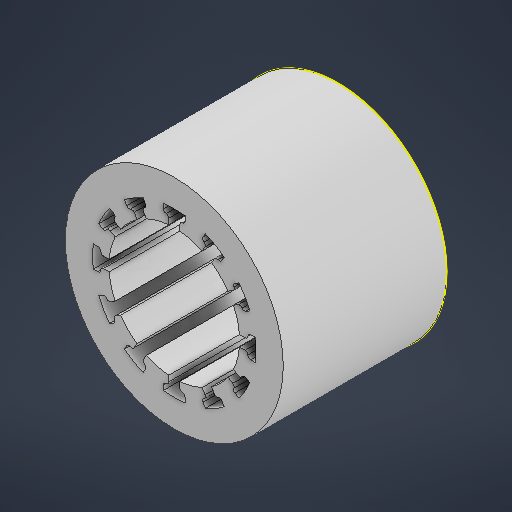
# Autodesk Inventor part: СИСЬКА
Saved by Autodesk Inventor 2025 (Build 290162000, 162)
## iProperties
Created: 2025-10-03
Part Number: СИСЬКА
Material: Типовые
Document SubType Name: Modeling
Designer: Phantom
Density: 1 g/cm^3
Appearance: По умолчанию
Author: Phantom
Autodesk Inventor part; units mm, degrees
ref_plane "YZ Plane" through (0, 0, 0) normal (1, 0, 0) x (0, 1, 0)
ref_plane "XZ Plane" through (0, 0, 0) normal (0, 1, 0) x (-1, 0, 0)
ref_plane "XY Plane" through (0, 0, 0) normal (0, 0, 1) x (1, 0, 0)
sketch "Эскиз1" plane through (0, 0, 0) normal (0, 0, 1) x (1, 0, 0)
  line L0 (-10.0069, -9.9098) -> (-10.0069, 10.0902)
  line L1 (-10.0069, 10.0902) -> (9.9931, 10.0902)
  line L2 (9.9931, 10.0902) -> (9.9931, -9.9098)
  line L3 (9.9931, -9.9098) -> (-10.0069, -9.9098)
  arc A0 (15.9207, 25.1962) -> (15.3056, 28.1887) centre (14.3486, 26.4325) ccw
  line L4 (10.8274, 18.7196) -> (15.9207, 25.1962)
  arc A1 (8.4102, 18.1432) -> (10.8274, 18.7196) centre (9.2553, 19.9559) ccw
  arc A2 (8.4102, 18.1432) -> (6.3595, 18.9642) centre (-0.0069, 0.0902) ccw
  arc A3 (5.0078, 21.0494) -> (6.3595, 18.9642) centre (6.9987, 20.8593) ccw
  line L5 (5.791, 29.2515) -> (5.0078, 21.0494)
  arc A4 (8.3012, 30.9928) -> (5.791, 29.2515) centre (7.7819, 29.0614) ccw
  arc A5 (8.3012, 30.9928) -> (-2.3164, 32.0067) centre (-0.0069, 0.0902) ccw
  arc A6 (-0.1811, 29.8218) -> (-2.3164, 32.0067) centre (-2.1721, 30.0119) ccw
  line L6 (-0.9643, 21.6197) -> (-0.1811, 29.8218)
  arc A7 (-2.6862, 19.828) -> (-0.9643, 21.6197) centre (-2.9553, 21.8098) ccw
  arc A8 (-2.6862, 19.828) -> (-4.8552, 19.4099) centre (-0.0069, 0.0902) ccw
  arc A9 (-7.1197, 20.4333) -> (-4.8552, 19.4099) centre (-5.342, 21.3498) ccw
  line L7 (-10.8952, 27.7568) -> (-7.1197, 20.4333)
  arc A10 (-9.7249, 30.5788) -> (-10.8952, 27.7568) centre (-9.1176, 28.6733) ccw
  arc A11 (-9.7249, 30.5788) -> (-19.2052, 25.6914) centre (-0.0069, 0.0902) ccw
  arc A12 (-16.2276, 25.0078) -> (-19.2052, 25.6914) centre (-18.0053, 24.0914) ccw
  line L8 (-12.4521, 17.6843) -> (-16.2276, 25.0078)
  arc A13 (-12.932, 15.2461) -> (-12.4521, 17.6843) centre (-14.2297, 16.7678) ccw
  arc A14 (-12.932, 15.2461) -> (-14.5306, 13.7218) centre (-0.0069, 0.0902) ccw
  arc A15 (-16.9889, 13.3584) -> (-14.5306, 13.7218) centre (-15.9889, 15.0905) ccw
  line L9 (-24.1245, 17.4781) -> (-16.9889, 13.3584)
  arc A16 (-24.6657, 20.4849) -> (-24.1245, 17.4781) centre (-23.1245, 19.2102) ccw
  arc A17 (-24.6657, 20.4849) -> (-29.9986, 11.2479) centre (-0.0069, 0.0902) ccw
  arc A18 (-27.1241, 12.2826) -> (-29.9986, 11.2479) centre (-28.1241, 10.5506) ccw
  line L10 (-19.9885, 8.1629) -> (-27.1241, 12.2826)
  arc A19 (-19.0741, 5.8523) -> (-19.9885, 8.1629) centre (-20.9885, 6.4309) ccw
  arc A20 (-19.0741, 5.8523) -> (-19.5948, 3.7057) centre (-0.0069, 0.0902) ccw
  arc A21 (-21.4664, 2.0709) -> (-19.5948, 3.7057) centre (-21.5616, 4.0687) ccw
  line L11 (-29.6965, 1.6789) -> (-21.4664, 2.0709)
  arc A22 (-31.7774, 3.9157) -> (-29.6965, 1.6789) centre (-29.7917, 3.6766) ccw
  arc A23 (-31.7774, 3.9157) -> (-31.2699, -6.7381) centre (-0.0069, 0.0902) ccw
  arc A24 (-29.4111, -4.3136) -> (-31.2699, -6.7381) centre (-29.3159, -6.3113) ccw
  line L12 (-21.181, -3.9215) -> (-29.4111, -4.3136)
  arc A25 (-19.1625, -5.3709) -> (-21.181, -3.9215) centre (-21.0858, -5.9193) ccw
  arc A26 (-19.1625, -5.3709) -> (-18.44, -7.4583) centre (-0.0069, 0.0902) ccw
  arc A27 (-19.1307, -9.8454) -> (-18.44, -7.4583) centre (-20.2908, -8.2163) ccw
  line L13 (-25.8424, -14.6248) -> (-19.1307, -9.8454)
  arc A28 (-28.8022, -13.868) -> (-25.8424, -14.6248) centre (-27.0025, -12.9956) ccw
  arc A29 (-28.8022, -13.868) -> (-22.6154, -22.5562) centre (-0.0069, 0.0902) ccw
  arc A30 (-22.3624, -19.5116) -> (-22.6154, -22.5562) centre (-21.2023, -21.1408) ccw
  line L14 (-15.6508, -14.7323) -> (-22.3624, -19.5116)
  arc A31 (-13.1691, -14.8603) -> (-15.6508, -14.7323) centre (-14.4907, -16.3614) ccw
  arc A32 (-13.1691, -14.8603) -> (-11.4328, -16.2257) centre (-0.0069, 0.0902) ccw
  arc A33 (-10.7233, -18.6073) -> (-11.4328, -16.2257) centre (-12.58, -17.864) ccw
  line L15 (-13.7856, -26.2565) -> (-10.7233, -18.6073)
  arc A34 (-16.6847, -27.2201) -> (-13.7856, -26.2565) centre (-15.6423, -25.5132) ccw
  arc A35 (-16.6847, -27.2201) -> (-6.7828, -31.1842) centre (-0.0069, 0.0902) ccw
  arc A36 (-8.2161, -28.4862) -> (-6.7828, -31.1842) centre (-6.3593, -29.2296) ccw
  line L16 (-5.1538, -20.837) -> (-8.2161, -28.4862)
  arc A37 (-2.9968, -19.603) -> (-5.1538, -20.837) centre (-3.297, -21.5803) ccw
  arc A38 (-2.9968, -19.603) -> (-0.7979, -19.813) centre (-0.0069, 0.0902) ccw
  arc A39 (1.0865, -21.4329) -> (-0.7979, -19.813) centre (-0.8773, -21.8114) ccw
  line L17 (2.6459, -29.5234) -> (1.0865, -21.4329)
  arc A40 (0.7279, -31.9014) -> (2.6459, -29.5234) centre (0.682, -29.9019) ccw
  arc A41 (0.7279, -31.9014) -> (11.201, -29.8829) centre (-0.0069, 0.0902) ccw
  arc A42 (8.5367, -28.3881) -> (11.201, -29.8829) centre (10.5006, -28.0096) ccw
  line L18 (6.9789, -20.3054) -> (8.5367, -28.3881)
  arc A43 (8.1187, -18.1045) -> (6.9789, -20.3054) centre (8.9427, -19.9268) ccw
  arc A44 (8.1187, -18.1045) -> (10.086, -17.0832) centre (-0.3176, 0.5517) ccw
  arc A45 (12.5497, -17.4256) -> (10.086, -17.0832) centre (11.1023, -18.8058) ccw
  line L19 (18.2351, -23.3882) -> (12.5497, -17.4256)
  arc A46 (17.9072, -26.4256) -> (18.2351, -23.3882) centre (16.7876, -24.7684) ccw
  arc A47 (17.9072, -26.4256) -> (25.6265, -19.0653) centre (-0.0069, 0.0902) ccw
  arc A48 (22.5769, -19.2482) -> (25.6265, -19.0653) centre (24.0244, -17.8681) ccw
  line L20 (16.8911, -13.2851) -> (22.5769, -19.2482)
  arc A49 (16.6646, -10.8104) -> (16.8911, -13.2851) centre (18.3385, -11.9049) ccw
  arc A50 (16.6646, -10.8104) -> (17.769, -8.8975) centre (-0.0069, 0.0902) ccw
  arc A51 (20.0254, -7.8563) -> (17.769, -8.8975) centre (19.5539, -9.7999) ccw
  line L21 (28.0326, -9.7988) -> (20.0254, -7.8563)
  arc A52 (29.3989, -12.5312) -> (28.0326, -9.7988) centre (27.5611, -11.7424) ccw
  arc A53 (29.3989, -12.5312) -> (31.9135, -2.166) centre (-0.0069, 0.0902) ccw
  arc A54 (29.447, -3.9686) -> (31.9135, -2.166) centre (29.9185, -2.025) ccw
  line L22 (21.4398, -2.0261) -> (29.447, -3.9686)
  arc A55 (19.9114, -0.0667) -> (21.4398, -2.0261) centre (21.9113, -0.0825) ccw
  arc A56 (19.9114, -0.0667) -> (19.8062, 2.1397) centre (-0.0069, 0.0902) ccw
  arc A57 (21.1415, 4.2355) -> (19.8062, 2.1397) centre (21.7956, 2.3455) ccw
  line L23 (28.9278, 6.9303) -> (21.1415, 4.2355)
  arc A58 (31.5545, 5.3703) -> (28.9278, 6.9303) centre (29.5819, 5.0403) ccw
  arc A59 (31.5545, 5.3703) -> (23.2125, 22.1098) centre (-0.0069, 0.0902) ccw
  arc A60 (26.9459, 12.7815) -> (28.2217, 15.1615) centre (26.2834, 14.6686) ccw
  line L24 (19.1717, 10.0522) -> (26.9459, 12.7815)
  arc A61 (16.8229, 10.8638) -> (19.1717, 10.0522) centre (18.5092, 11.9393) ccw
  arc A62 (16.8229, 10.8638) -> (15.5337, 12.6575) centre (0.0291, 0.1528) ccw
  arc A63 (15.5129, 15.1424) -> (15.5337, 12.6575) centre (17.0905, 13.913) ccw
  line L25 (20.5775, 21.6415) -> (15.5129, 15.1424)
  arc A64 (23.2125, 22.1098) -> (20.5775, 21.6415) centre (22.155, 20.4122) ccw
  arc A65 (23.2125, 22.1098) -> (15.3056, 28.1887) centre (-0.0069, 0.0902) ccw
  arc A66 (8.4102, 18.1432) -> (6.3595, 18.9642) centre (-0.0069, 0.0902) ccw
  arc A67 (8.4102, 18.1432) -> (10.8274, 18.7196) centre (9.2553, 19.9559) ccw
  line L26 (10.8274, 18.7196) -> (15.9207, 25.1962)
  arc A68 (15.9207, 25.1962) -> (15.3056, 28.1887) centre (14.3486, 26.4325) ccw
  arc A69 (15.3056, 28.1887) -> (8.3012, 30.9928) centre (-0.0069, 0.0902) ccw
  arc A70 (8.3012, 30.9928) -> (5.791, 29.2515) centre (7.7819, 29.0614) ccw
  line L27 (5.791, 29.2515) -> (5.0078, 21.0494)
  arc A71 (5.0078, 21.0494) -> (6.3595, 18.9642) centre (6.9987, 20.8593) ccw
  line L28 (-0.9643, 21.6197) -> (-0.1811, 29.8218)
  arc A72 (-0.1811, 29.8218) -> (-2.3164, 32.0067) centre (-2.1721, 30.0119) ccw
  arc A73 (-2.3164, 32.0067) -> (-9.7249, 30.5788) centre (-0.0069, 0.0902) ccw
  arc A74 (-9.7249, 30.5788) -> (-10.8952, 27.7568) centre (-9.1176, 28.6733) ccw
  line L29 (-10.8952, 27.7568) -> (-7.1197, 20.4333)
  arc A75 (-7.1197, 20.4333) -> (-4.8552, 19.4099) centre (-5.342, 21.3498) ccw
  arc A76 (-2.6862, 19.828) -> (-4.8552, 19.4099) centre (-0.0069, 0.0902) ccw
  arc A77 (-2.6862, 19.828) -> (-0.9643, 21.6197) centre (-2.9553, 21.8098) ccw
  arc A78 (-12.932, 15.2461) -> (-14.5306, 13.7218) centre (-0.0069, 0.0902) ccw
  arc A79 (-12.932, 15.2461) -> (-12.4521, 17.6843) centre (-14.2297, 16.7678) ccw
  line L30 (-12.4521, 17.6843) -> (-16.2276, 25.0078)
  arc A80 (-16.2276, 25.0078) -> (-19.2052, 25.6914) centre (-18.0053, 24.0914) ccw
  arc A81 (-19.2052, 25.6914) -> (-24.6657, 20.4849) centre (-0.0069, 0.0902) ccw
  arc A82 (-24.6657, 20.4849) -> (-24.1245, 17.4781) centre (-23.1245, 19.2102) ccw
  line L31 (-24.1245, 17.4781) -> (-16.9889, 13.3584)
  arc A83 (-16.9889, 13.3584) -> (-14.5306, 13.7218) centre (-15.9889, 15.0905) ccw
  arc A84 (-29.9986, 11.2479) -> (-31.7774, 3.9157) centre (-0.0069, 0.0902) ccw
  arc A85 (-31.7774, 3.9157) -> (-29.6965, 1.6789) centre (-29.7917, 3.6766) ccw
  line L32 (-29.6965, 1.6789) -> (-21.4664, 2.0709)
  arc A86 (-21.4664, 2.0709) -> (-19.5948, 3.7057) centre (-21.5616, 4.0687) ccw
  arc A87 (-19.0741, 5.8523) -> (-19.5948, 3.7057) centre (-0.0069, 0.0902) ccw
  arc A88 (-19.0741, 5.8523) -> (-19.9885, 8.1629) centre (-20.9885, 6.4309) ccw
  line L33 (-19.9885, 8.1629) -> (-27.1241, 12.2826)
  arc A89 (-27.1241, 12.2826) -> (-29.9986, 11.2479) centre (-28.1241, 10.5506) ccw
  arc A90 (-31.2699, -6.7381) -> (-28.8022, -13.868) centre (-0.0069, 0.0902) ccw
  arc A91 (-28.8022, -13.868) -> (-25.8424, -14.6248) centre (-27.0025, -12.9956) ccw
  line L34 (-25.8424, -14.6248) -> (-19.1307, -9.8454)
  arc A92 (-19.1307, -9.8454) -> (-18.44, -7.4583) centre (-20.2908, -8.2163) ccw
  arc A93 (-19.1625, -5.3709) -> (-18.44, -7.4583) centre (-0.0069, 0.0902) ccw
  arc A94 (-19.1625, -5.3709) -> (-21.181, -3.9215) centre (-21.0858, -5.9193) ccw
  line L35 (-21.181, -3.9215) -> (-29.4111, -4.3136)
  arc A95 (-29.4111, -4.3136) -> (-31.2699, -6.7381) centre (-29.3159, -6.3113) ccw
  arc A96 (-6.7828, -31.1842) -> (0.7279, -31.9014) centre (-0.0069, 0.0902) ccw
  arc A97 (0.7279, -31.9014) -> (2.6459, -29.5234) centre (0.682, -29.9019) ccw
  line L36 (2.6459, -29.5234) -> (1.0865, -21.4329)
  arc A98 (1.0865, -21.4329) -> (-0.7979, -19.813) centre (-0.8773, -21.8114) ccw
  arc A99 (-2.9968, -19.603) -> (-0.7979, -19.813) centre (-0.0069, 0.0902) ccw
  arc A100 (-2.9968, -19.603) -> (-5.1538, -20.837) centre (-3.297, -21.5803) ccw
  line L37 (-5.1538, -20.837) -> (-8.2161, -28.4862)
  arc A101 (-8.2161, -28.4862) -> (-6.7828, -31.1842) centre (-6.3593, -29.2296) ccw
  arc A102 (11.201, -29.8829) -> (17.9072, -26.4256) centre (-0.0069, 0.0902) ccw
  arc A103 (17.9072, -26.4256) -> (18.2351, -23.3882) centre (16.7876, -24.7684) ccw
  line L38 (18.2351, -23.3882) -> (12.5497, -17.4256)
  arc A104 (12.5497, -17.4256) -> (10.086, -17.0832) centre (11.1023, -18.8058) ccw
  arc A105 (8.1187, -18.1045) -> (10.086, -17.0832) centre (-0.3176, 0.5517) ccw
  arc A106 (8.1187, -18.1045) -> (6.9789, -20.3054) centre (8.9427, -19.9268) ccw
  line L39 (6.9789, -20.3054) -> (8.5367, -28.3881)
  arc A107 (8.5367, -28.3881) -> (11.201, -29.8829) centre (10.5006, -28.0096) ccw
  arc A108 (-22.6154, -22.5562) -> (-16.6847, -27.2201) centre (-0.0069, 0.0902) ccw
  arc A109 (-16.6847, -27.2201) -> (-13.7856, -26.2565) centre (-15.6423, -25.5132) ccw
  line L40 (-13.7856, -26.2565) -> (-10.7233, -18.6073)
  arc A110 (-10.7233, -18.6073) -> (-11.4328, -16.2257) centre (-12.58, -17.864) ccw
  arc A111 (-13.1691, -14.8603) -> (-11.4328, -16.2257) centre (-0.0069, 0.0902) ccw
  arc A112 (-13.1691, -14.8603) -> (-15.6508, -14.7323) centre (-14.4907, -16.3614) ccw
  line L41 (-15.6508, -14.7323) -> (-22.3624, -19.5116)
  arc A113 (-22.3624, -19.5116) -> (-22.6154, -22.5562) centre (-21.2023, -21.1408) ccw
  arc A114 (16.6646, -10.8104) -> (17.769, -8.8975) centre (-0.0069, 0.0902) ccw
  arc A115 (16.6646, -10.8104) -> (16.8911, -13.2851) centre (18.3385, -11.9049) ccw
  line L42 (16.8911, -13.2851) -> (22.5769, -19.2482)
  arc A116 (22.5769, -19.2482) -> (25.6265, -19.0653) centre (24.0244, -17.8681) ccw
  arc A117 (25.6265, -19.0653) -> (29.3989, -12.5312) centre (-0.0069, 0.0902) ccw
  arc A118 (29.3989, -12.5312) -> (28.0326, -9.7988) centre (27.5611, -11.7424) ccw
  line L43 (28.0326, -9.7988) -> (20.0254, -7.8563)
  arc A119 (20.0254, -7.8563) -> (17.769, -8.8975) centre (19.5539, -9.7999) ccw
  line L44 (21.4398, -2.0261) -> (29.447, -3.9686)
  arc A120 (29.447, -3.9686) -> (31.9135, -2.166) centre (29.9185, -2.025) ccw
  arc A121 (31.9135, -2.166) -> (31.5545, 5.3703) centre (-0.0069, 0.0902) ccw
  arc A122 (31.5545, 5.3703) -> (28.9278, 6.9303) centre (29.5819, 5.0403) ccw
  line L45 (28.9278, 6.9303) -> (21.1415, 4.2355)
  arc A123 (21.1415, 4.2355) -> (19.8062, 2.1397) centre (21.7956, 2.3455) ccw
  arc A124 (19.9114, -0.0667) -> (19.8062, 2.1397) centre (-0.0069, 0.0902) ccw
  arc A125 (19.9114, -0.0667) -> (21.4398, -2.0261) centre (21.9113, -0.0825) ccw
  circle A126 centre (-0.0069, 0.0902) radius 40
  point P0 (0, 0)
  point P1 (-1.2221, -0.4307)
  point P2 (15.3056, 28.1887)
  point P3 (5.0078, 21.0494)
  point P4 (-2.3164, 32.0067)
  point P5 (-4.8552, 19.4099)
  point P6 (-7.1197, 20.4333)
  point P7 (-9.7249, 30.5788)
  point P8 (-16.9889, 13.3584)
  point P9 (-31.7774, 3.9157)
  point P10 (-31.2699, -6.7381)
  point P11 (-28.8022, -13.868)
  point P12 (-22.6154, -22.5562)
  point P13 (-6.7828, -31.1842)
  point P14 (0.7279, -31.9014)
  point P15 (11.201, -29.8829)
  point P16 (17.9072, -26.4256)
  point P17 (21.4398, -2.0261)
  dimension "d0" = 80
  constraints: 253 point on circle, 127 centre point, 92 end point, 1 coincident
  measures "d0" diameter of A126
extrude "Выдавливание1" add sketch "Эскиз1" along normal blind 60 contours L4 A1 A2 A3 L5 A4 A69 A0 | A0 A65 A64 L25 A63 A62 A61 L24 A60 A59 A58 L23 A57 A56 A55 L22 A54 A53 A52 L21 A51 A50 A49 L20 A48 A47 A46 L19 A45 A44 A43 L18 A42 A41 A40 L17 A39 A38 A37 L16 A36 A35 A34 L15 A33 A32 A31 L14 A30 A29 A28 L13 A27 A26 A25 L12 A24 A23 A22 L11 A21 A20 A19 L10 A18 A17 A16 L9 A15 A14 A13 L8 A12 A11 A10 L7 A9 A8 A7 L6 A6 A5 A4 L5 A3 A2 A1 L4 | A59 A60 L24 A61 A62 A63 L25 A64 | A6 L6 A7 A8 A9 L7 A10 A73 | A121 A54 L22 A55 A56 A57 L23 A58 | A12 L8 A13 A14 A15 L9 A16 A81 | A117 A48 L20 A49 A50 A51 L21 A52 | A18 L10 A19 A20 A21 L11 A22 A84 | A102 A42 L18 A43 A44 A45 L19 A46 | A24 L12 A25 A26 A27 L13 A28 A90 | A96 A36 L16 A37 A38 A39 L17 A40 | A30 L14 A31 A32 A33 L15 A34 A108 | A126
sketch "Эскиз4" plane through (-0.0069, 0.0902, 60) normal (0, 0, 1) x (1, 0, 0)
  circle A0 centre (0, 0) radius 40 projected
  circle A1 centre (0, 0) radius 30
  line L0 (0, 30) -> (0, -30)
  line L1 (-4, 30) -> (-4, 28)
  line L2 (4, 30) -> (4, 28)
  line L3 (3, 27) -> (3, 27)
  line L4 (-2, 26) -> (-2, -30)
  line L5 (2, 26) -> (2, -30)
  arc A2 (-2, 26) -> (-3, 27) centre (-3, 26) ccw
  arc A3 (-4, 28) -> (-3, 27) centre (-3, 28) ccw
  arc A4 (3, 27) -> (4, 28) centre (3, 28) ccw
  arc A5 (3, 27) -> (2, 26) centre (3, 26) ccw
  line L6 (-4, 34.038) -> (4, 34.038)
  circle A6 centre (0, 0) radius 24
  line L7 (-18.4641, 23.9808) -> (-17.4641, 22.2487)
  arc A7 (-17.4641, 22.2487) -> (-16.0981, 21.8827) centre (-16.5981, 22.7487) ccw
  arc A8 (-14.7321, 21.5167) -> (-16.0981, 21.8827) centre (-15.5981, 21.0167) ccw
  line L8 (-14.7321, 21.5167) -> (13.2679, -26.9808)
  line L9 (-11.2679, 23.5167) -> (16.7321, -24.9808)
  arc A9 (-10.9019, 24.8827) -> (-11.2679, 23.5167) centre (-10.4019, 24.0167) ccw
  arc A10 (-10.9019, 24.8827) -> (-10.5359, 26.2487) centre (-11.4019, 25.7487) ccw
  line L10 (-11.5359, 27.9808) -> (-10.5359, 26.2487)
  line L11 (-27.9808, 11.5359) -> (-26.2487, 10.5359)
  arc A11 (-26.2487, 10.5359) -> (-24.8827, 10.9019) centre (-25.7487, 11.4019) ccw
  arc A12 (-23.5167, 11.2679) -> (-24.8827, 10.9019) centre (-24.0167, 10.4019) ccw
  line L12 (-23.5167, 11.2679) -> (24.9808, -16.7321)
  line L13 (-21.5167, 14.7321) -> (26.9808, -13.2679)
  arc A13 (-21.8827, 16.0981) -> (-21.5167, 14.7321) centre (-21.0167, 15.5981) ccw
  arc A14 (-21.8827, 16.0981) -> (-22.2487, 17.4641) centre (-22.7487, 16.5981) ccw
  line L14 (-23.9808, 18.4641) -> (-22.2487, 17.4641)
  line L15 (-30, -4) -> (-28, -4)
  arc A15 (-28, -4) -> (-27, -3) centre (-28, -3) ccw
  arc A16 (-26, -2) -> (-27, -3) centre (-26, -3) ccw
  line L16 (-26, -2) -> (30, -2)
  line L17 (-26, 2) -> (30, 2)
  arc A17 (-27, 3) -> (-26, 2) centre (-26, 3) ccw
  arc A18 (-27, 3) -> (-28, 4) centre (-28, 3) ccw
  line L18 (-30, 4) -> (-28, 4)
  line L19 (-23.9808, -18.4641) -> (-22.2487, -17.4641)
  arc A19 (-22.2487, -17.4641) -> (-21.8827, -16.0981) centre (-22.7487, -16.5981) ccw
  arc A20 (-21.5167, -14.7321) -> (-21.8827, -16.0981) centre (-21.0167, -15.5981) ccw
  line L20 (-21.5167, -14.7321) -> (26.9808, 13.2679)
  line L21 (-23.5167, -11.2679) -> (24.9808, 16.7321)
  arc A21 (-24.8827, -10.9019) -> (-23.5167, -11.2679) centre (-24.0167, -10.4019) ccw
  arc A22 (-24.8827, -10.9019) -> (-26.2487, -10.5359) centre (-25.7487, -11.4019) ccw
  line L22 (-27.9808, -11.5359) -> (-26.2487, -10.5359)
  line L23 (-11.5359, -27.9808) -> (-10.5359, -26.2487)
  arc A23 (-10.5359, -26.2487) -> (-10.9019, -24.8827) centre (-11.4019, -25.7487) ccw
  arc A24 (-11.2679, -23.5167) -> (-10.9019, -24.8827) centre (-10.4019, -24.0167) ccw
  line L24 (-11.2679, -23.5167) -> (16.7321, 24.9808)
  line L25 (-14.7321, -21.5167) -> (13.2679, 26.9808)
  arc A25 (-16.0981, -21.8827) -> (-14.7321, -21.5167) centre (-15.5981, -21.0167) ccw
  arc A26 (-16.0981, -21.8827) -> (-17.4641, -22.2487) centre (-16.5981, -22.7487) ccw
  line L26 (-18.4641, -23.9808) -> (-17.4641, -22.2487)
  line L27 (4, -30) -> (4, -28)
  arc A27 (4, -28) -> (3, -27) centre (3, -28) ccw
  arc A28 (2, -26) -> (3, -27) centre (3, -26) ccw
  line L28 (2, -26) -> (2, 30)
  line L29 (-2, -26) -> (-2, 30)
  arc A29 (-3, -27) -> (-2, -26) centre (-3, -26) ccw
  arc A30 (-3, -27) -> (-4, -28) centre (-3, -28) ccw
  line L30 (-4, -30) -> (-4, -28)
  line L31 (18.4641, -23.9808) -> (17.4641, -22.2487)
  arc A31 (17.4641, -22.2487) -> (16.0981, -21.8827) centre (16.5981, -22.7487) ccw
  arc A32 (14.7321, -21.5167) -> (16.0981, -21.8827) centre (15.5981, -21.0167) ccw
  line L32 (14.7321, -21.5167) -> (-13.2679, 26.9808)
  line L33 (11.2679, -23.5167) -> (-16.7321, 24.9808)
  arc A33 (10.9019, -24.8827) -> (11.2679, -23.5167) centre (10.4019, -24.0167) ccw
  arc A34 (10.9019, -24.8827) -> (10.5359, -26.2487) centre (11.4019, -25.7487) ccw
  line L34 (11.5359, -27.9808) -> (10.5359, -26.2487)
  line L35 (27.9808, -11.5359) -> (26.2487, -10.5359)
  arc A35 (26.2487, -10.5359) -> (24.8827, -10.9019) centre (25.7487, -11.4019) ccw
  arc A36 (23.5167, -11.2679) -> (24.8827, -10.9019) centre (24.0167, -10.4019) ccw
  line L36 (23.5167, -11.2679) -> (-24.9808, 16.7321)
  line L37 (21.5167, -14.7321) -> (-26.9808, 13.2679)
  arc A37 (21.8827, -16.0981) -> (21.5167, -14.7321) centre (21.0167, -15.5981) ccw
  arc A38 (21.8827, -16.0981) -> (22.2487, -17.4641) centre (22.7487, -16.5981) ccw
  line L38 (23.9808, -18.4641) -> (22.2487, -17.4641)
  line L39 (30, 4) -> (28, 4)
  arc A39 (28, 4) -> (27, 3) centre (28, 3) ccw
  arc A40 (26, 2) -> (27, 3) centre (26, 3) ccw
  line L40 (26, 2) -> (-30, 2)
  line L41 (26, -2) -> (-30, -2)
  arc A41 (27, -3) -> (26, -2) centre (26, -3) ccw
  arc A42 (27, -3) -> (28, -4) centre (28, -3) ccw
  line L42 (30, -4) -> (28, -4)
  line L43 (23.9808, 18.4641) -> (22.2487, 17.4641)
  arc A43 (22.2487, 17.4641) -> (21.8827, 16.0981) centre (22.7487, 16.5981) ccw
  arc A44 (21.5167, 14.7321) -> (21.8827, 16.0981) centre (21.0167, 15.5981) ccw
  line L44 (21.5167, 14.7321) -> (-26.9808, -13.2679)
  line L45 (23.5167, 11.2679) -> (-24.9808, -16.7321)
  arc A45 (24.8827, 10.9019) -> (23.5167, 11.2679) centre (24.0167, 10.4019) ccw
  arc A46 (24.8827, 10.9019) -> (26.2487, 10.5359) centre (25.7487, 11.4019) ccw
  line L46 (27.9808, 11.5359) -> (26.2487, 10.5359)
  line L47 (11.5359, 27.9808) -> (10.5359, 26.2487)
  arc A47 (10.5359, 26.2487) -> (10.9019, 24.8827) centre (11.4019, 25.7487) ccw
  arc A48 (11.2679, 23.5167) -> (10.9019, 24.8827) centre (10.4019, 24.0167) ccw
  line L48 (11.2679, 23.5167) -> (-16.7321, -24.9808)
  line L49 (14.7321, 21.5167) -> (-13.2679, -26.9808)
  arc A49 (16.0981, 21.8827) -> (14.7321, 21.5167) centre (15.5981, 21.0167) ccw
  arc A50 (16.0981, 21.8827) -> (17.4641, 22.2487) centre (16.5981, 22.7487) ccw
  line L50 (18.4641, 23.9808) -> (17.4641, 22.2487)
  point P0 (-20.4831, 27.4778)
  point P1 (-31.4778, 13.5549)
  point P2 (-34.038, -4)
  point P3 (-27.4778, -20.4831)
  point P4 (-13.5549, -31.4778)
  point P5 (4, -34.038)
  point P6 (20.4831, -27.4778)
  point P7 (31.4778, -13.5549)
  point P8 (34.038, 4)
  point P9 (27.4778, 20.4831)
  point P10 (13.5549, 31.4778)
  point P11 (-13.6903, 19.7123)
  point P12 (-10.2262, 21.7123)
  point P13 (-10.9019, 24.8827)
  point P14 (-11.402, 27.7488)
  point P15 (-18.3302, 23.7488)
  point P16 (4, 29.7321)
  point P17 (-4, 29.7321)
  point P18 (-2, 23.9165)
  point P19 (2, 23.9165)
  point P20 (16.0981, 21.8827)
  point P21 (18.3302, 23.7488)
  point P22 (11.402, 27.7488)
  point P23 (10.2262, 21.7123)
  point P24 (13.6903, 19.7123)
  point P25 (21.5167, 14.7321)
  point P26 (19.7123, 13.6903)
  point P27 (21.7123, 10.2262)
  point P28 (24.8827, 10.9019)
  point P29 (27.7488, 11.402)
  point P30 (23.7488, 18.3302)
  point P31 (23.9165, 2)
  point P32 (23.9165, -2)
  point P33 (29.7321, -4)
  point P34 (29.7321, 4)
  point P35 (23.7488, -18.3302)
  point P36 (27.7488, -11.402)
  point P37 (23.5167, -11.2679)
  point P38 (21.7123, -10.2262)
  point P39 (19.7123, -13.6903)
  point P40 (10.9019, -24.8827)
  point P41 (11.402, -27.7488)
  point P42 (18.3302, -23.7488)
  point P43 (13.6903, -19.7123)
  point P44 (10.2262, -21.7123)
  point P45 (-2, -23.9165)
  point P46 (-4, -29.7321)
  point P47 (4, -29.7321)
  point P48 (2, -23.9165)
  point P49 (-10.2262, -21.7123)
  point P50 (-13.6903, -19.7123)
  point P51 (-18.3302, -23.7488)
  point P52 (-11.402, -27.7488)
  point P53 (-19.7123, -13.6903)
  point P54 (-21.7123, -10.2262)
  point P55 (-24.8827, -10.9019)
  point P56 (-27.7488, -11.402)
  point P57 (-23.7488, -18.3302)
  point P58 (-23.9165, -2)
  point P59 (-23.9165, 2)
  point P60 (-29.7321, 4)
  point P61 (-29.7321, -4)
  point P62 (-21.7123, 10.2262)
  point P63 (-19.7123, 13.6903)
  point P64 (-23.7488, 18.3302)
  point P65 (-27.7488, 11.402)
  dimension "d7" = 60
  dimension "d15" = 48
  dimension "d8" = 4
  dimension "d9" = 4
  dimension "d10" = 3
  dimension "d11" = 2
  dimension "d12" = 2
  dimension "d13" = 1
  dimension "d14" = 1
  dimension "d18" = 360
  constraints: 102 end point, 96 point on circle, 48 centre point, 12 point on line, 8 tangent, 4 parallel, 2 coincident, 2 equal radius, 2 horizontal, 1 vertical, 295 other
  measures "d8" distance between parallel lines of L0 L1
  measures "d9" distance between parallel lines of L0 L2
  measures "d10" distance from line of L0.start L3
  measures "d11" distance between parallel lines of L0 L4
  measures "d12" distance between parallel lines of L0 L5
  measures "d13" radius of A2
  measures "d14" radius of A4
extrude "Выдавливание3" cut sketch "Эскиз4" against normal blind 60 contours A1 L16 A6 L17 | L17 A40 A39 L39 A1 | A1 L42 A42 A41 L16 | L46 A46 A45 L20 A1 | L17 L20 A6 | A6 L16 L13 L20 L17 | A1 L13 A36 A35 L35 | A6 L13 L16 | L20 A6 L21 A1 | L20 L17 L24 L21 A6 | L20 L13 L24 L17 | A1 L12 A6 L13 | A6 L12 L9 L16 L13 | L16 L9 L20 L13 | L21 A44 A43 L43 A1 | L21 L24 A6 | L24 L13 L5 L17 | L17 L5 L21 L24 | L20 L9 L24 L13 | A1 L38 A38 A37 L12 | A6 L9 L12 | L16 L5 L20 L9 | L9 L12 L5 L16 | L24 L21 L5 L25 A6 | A6 L25 A1 L24 | L17 L9 L21 L5 | L5 L13 L9 L17 | L24 L9 L5 L13 | L20 L5 L24 L9 | L9 A1 L8 A6 | A6 L8 L5 L12 L9 | L16 L24 L20 L5 | L5 L12 L24 L16 | L50 A50 A49 L24 A1 | L25 L5 A6 | L21 L9 L25 L5 | L5 L9 L13 | L17 L13 L21 L9 | L9 L13 L17 | L24 L5 L9 | L20 L24 L5 | A1 L9 A32 A31 L31 | A6 L5 L8 | L5 L8 L24 L12 | L24 L12 L20 L16 | L16 L20 L24 | A6 L0 A1 L28 L5 | L5 L25 L0 A6 | A48 A47 L47 A1 L25 | L21 L0 L9 | L5 L24 L20 L16 L0 L17 L13 L9 | L17 L0 L13 | A6 L0 L8 L5 | L5 A1 L0 A6 | L8 A1 L34 A34 A33 | L24 L0 L12 | L20 L0 L16 | L28 A1 L2 A4 A5 | A6 L4 L29 A1 L0 | L0 L9 L4 A6 | L25 L13 L4 L9 | L0 L13 L25 | L21 L17 L25 L13 | L0 L17 L21 | L0 L16 L12 L8 L4 L25 L21 L17 | A28 A27 L27 A1 L5 | A6 L4 L24 L0 | L0 A1 L4 A6 | L8 L20 L0 | L24 L4 L20 L8 | L12 L16 L0 | L20 L8 L16 L12 | L4 L9 A6 | L4 L13 L8 A6 L9 | L25 L17 L4 L13 | L21 L25 L17 | A6 L24 L4 | L20 L4 L16 L8 | L24 A6 L25 L20 L4 | L16 L8 L12 | L29 A2 A3 L1 A1 | A6 L8 L33 A1 L32 L9 | L4 L17 L8 L13 | L25 L21 L4 L17 | L25 L4 L21 | A1 L30 A30 A29 L4 | L24 L49 A1 L48 L25 A6 | L16 L4 L12 L8 | L20 L25 L16 L4 | L12 L4 L8 | L8 L13 A6 | L32 A1 L10 A10 A9 | L4 L21 L8 L17 | L8 L17 L12 A6 L13 | L4 L25 L8 L21 | L4 L8 L25 | A6 L20 L25 | A24 A23 L23 A1 L49 | L16 L25 L12 L4 | L20 A6 L21 L16 L25 | L4 L12 L25 L8 | A6 L12 L37 A1 L36 L13 | A8 A7 L7 A1 L33 | L8 L21 L12 L17 | L8 L25 L12 L21 | L20 L45 A1 L44 L21 A6 | L48 A1 L26 A26 A25 | L16 L21 L12 L25 | L12 L17 A6 | L36 A1 L14 A14 A13 | L12 L21 L16 A6 L17 | A6 L16 L21 | A20 A19 L19 A1 L45 | A6 L16 L41 A1 L40 L17 | A12 A11 L11 A1 L37 | L44 A1 L22 A22 A21 | L40 A1 L18 A18 A17 | A16 A15 L15 A1 L41
sketch "Эскиз5" plane through (-0.0069, 0.0902, 0) normal (0, 0, -1) x (-1, 0, 0)
  arc A0 (26, 2) -> (27, 3) centre (26, 3) ccw projected
  arc A1 (28, 4) -> (27, 3) centre (28, 3) ccw projected
  line L0 (28, 4) -> (29.7321, 4) projected
  arc A2 (29.7321, -4) -> (29.7321, 4) centre (0, 0) ccw projected
  line L1 (29.7321, -4) -> (28, -4) projected
  arc A3 (27, -3) -> (28, -4) centre (28, -3) ccw projected
  arc A4 (27, -3) -> (26, -2) centre (26, -3) ccw projected
  line L2 (26, -2) -> (23.9165, -2) projected
  arc A5 (21.7123, -10.2262) -> (23.9165, -2) centre (0, 0) ccw projected
  line L3 (21.7123, -10.2262) -> (23.5167, -11.2679) projected
  arc A6 (23.5167, -11.2679) -> (24.8827, -10.9019) centre (24.0167, -10.4019) ccw projected
  arc A7 (26.2487, -10.5359) -> (24.8827, -10.9019) centre (25.7487, -11.4019) ccw projected
  line L4 (26.2487, -10.5359) -> (27.7488, -11.402) projected
  arc A8 (23.7488, -18.3302) -> (27.7488, -11.402) centre (0, 0) ccw projected
  line L5 (23.7488, -18.3302) -> (22.2487, -17.4641) projected
  arc A9 (21.8827, -16.0981) -> (22.2487, -17.4641) centre (22.7487, -16.5981) ccw projected
  arc A10 (21.8827, -16.0981) -> (21.5167, -14.7321) centre (21.0167, -15.5981) ccw projected
  line L6 (21.5167, -14.7321) -> (19.7123, -13.6903) projected
  arc A11 (13.6903, -19.7123) -> (19.7123, -13.6903) centre (0, 0) ccw projected
  line L7 (13.6903, -19.7123) -> (14.7321, -21.5167) projected
  arc A12 (14.7321, -21.5167) -> (16.0981, -21.8827) centre (15.5981, -21.0167) ccw projected
  arc A13 (17.4641, -22.2487) -> (16.0981, -21.8827) centre (16.5981, -22.7487) ccw projected
  line L8 (17.4641, -22.2487) -> (18.3302, -23.7488) projected
  arc A14 (11.402, -27.7488) -> (18.3302, -23.7488) centre (0, 0) ccw projected
  line L9 (11.402, -27.7488) -> (10.5359, -26.2487) projected
  arc A15 (10.9019, -24.8827) -> (10.5359, -26.2487) centre (11.4019, -25.7487) ccw projected
  arc A16 (10.9019, -24.8827) -> (11.2679, -23.5167) centre (10.4019, -24.0167) ccw projected
  line L10 (11.2679, -23.5167) -> (10.2262, -21.7123) projected
  arc A17 (2, -23.9165) -> (10.2262, -21.7123) centre (0, 0) ccw projected
  line L11 (2, -23.9165) -> (2, -26) projected
  arc A18 (2, -26) -> (3, -27) centre (3, -26) ccw projected
  arc A19 (4, -28) -> (3, -27) centre (3, -28) ccw projected
  line L12 (4, -28) -> (4, -29.7321) projected
  arc A20 (-4, -29.7321) -> (4, -29.7321) centre (0, 0) ccw projected
  line L13 (-4, -29.7321) -> (-4, -28) projected
  arc A21 (-3, -27) -> (-4, -28) centre (-3, -28) ccw projected
  arc A22 (-3, -27) -> (-2, -26) centre (-3, -26) ccw projected
  line L14 (-2, -26) -> (-2, -23.9165) projected
  arc A23 (-10.2262, -21.7123) -> (-2, -23.9165) centre (0, 0) ccw projected
  line L15 (-10.2262, -21.7123) -> (-11.2679, -23.5167) projected
  arc A24 (-11.2679, -23.5167) -> (-10.9019, -24.8827) centre (-10.4019, -24.0167) ccw projected
  arc A25 (-10.5359, -26.2487) -> (-10.9019, -24.8827) centre (-11.4019, -25.7487) ccw projected
  line L16 (-10.5359, -26.2487) -> (-11.402, -27.7488) projected
  arc A26 (-18.3302, -23.7488) -> (-11.402, -27.7488) centre (0, 0) ccw projected
  line L17 (-18.3302, -23.7488) -> (-17.4641, -22.2487) projected
  arc A27 (-16.0981, -21.8827) -> (-17.4641, -22.2487) centre (-16.5981, -22.7487) ccw projected
  arc A28 (-16.0981, -21.8827) -> (-14.7321, -21.5167) centre (-15.5981, -21.0167) ccw projected
  line L18 (-14.7321, -21.5167) -> (-13.6903, -19.7123) projected
  arc A29 (-19.7123, -13.6903) -> (-13.6903, -19.7123) centre (0, 0) ccw projected
  line L19 (-19.7123, -13.6903) -> (-21.5167, -14.7321) projected
  arc A30 (-21.5167, -14.7321) -> (-21.8827, -16.0981) centre (-21.0167, -15.5981) ccw projected
  arc A31 (-22.2487, -17.4641) -> (-21.8827, -16.0981) centre (-22.7487, -16.5981) ccw projected
  line L20 (-22.2487, -17.4641) -> (-23.7488, -18.3302) projected
  arc A32 (-27.7488, -11.402) -> (-23.7488, -18.3302) centre (0, 0) ccw projected
  line L21 (-27.7488, -11.402) -> (-26.2487, -10.5359) projected
  arc A33 (-24.8827, -10.9019) -> (-26.2487, -10.5359) centre (-25.7487, -11.4019) ccw projected
  arc A34 (-24.8827, -10.9019) -> (-23.5167, -11.2679) centre (-24.0167, -10.4019) ccw projected
  line L22 (-23.5167, -11.2679) -> (-21.7123, -10.2262) projected
  arc A35 (-23.9165, -2) -> (-21.7123, -10.2262) centre (0, 0) ccw projected
  line L23 (-23.9165, -2) -> (-26, -2) projected
  arc A36 (-26, -2) -> (-27, -3) centre (-26, -3) ccw projected
  arc A37 (-28, -4) -> (-27, -3) centre (-28, -3) ccw projected
  line L24 (-28, -4) -> (-29.7321, -4) projected
  arc A38 (-29.7321, 4) -> (-29.7321, -4) centre (0, 0) ccw projected
  line L25 (-29.7321, 4) -> (-28, 4) projected
  arc A39 (-27, 3) -> (-28, 4) centre (-28, 3) ccw projected
  arc A40 (-27, 3) -> (-26, 2) centre (-26, 3) ccw projected
  line L26 (-26, 2) -> (-23.9165, 2) projected
  arc A41 (-21.7123, 10.2262) -> (-23.9165, 2) centre (0, 0) ccw projected
  line L27 (-21.7123, 10.2262) -> (-23.5167, 11.2679) projected
  arc A42 (-23.5167, 11.2679) -> (-24.8827, 10.9019) centre (-24.0167, 10.4019) ccw projected
  arc A43 (-26.2487, 10.5359) -> (-24.8827, 10.9019) centre (-25.7487, 11.4019) ccw projected
  line L28 (-26.2487, 10.5359) -> (-27.7488, 11.402) projected
  arc A44 (-23.7488, 18.3302) -> (-27.7488, 11.402) centre (0, 0) ccw projected
  line L29 (-23.7488, 18.3302) -> (-22.2487, 17.4641) projected
  arc A45 (-21.8827, 16.0981) -> (-22.2487, 17.4641) centre (-22.7487, 16.5981) ccw projected
  arc A46 (-21.8827, 16.0981) -> (-21.5167, 14.7321) centre (-21.0167, 15.5981) ccw projected
  line L30 (-21.5167, 14.7321) -> (-19.7123, 13.6903) projected
  arc A47 (-13.6903, 19.7123) -> (-19.7123, 13.6903) centre (0, 0) ccw projected
  line L31 (-13.6903, 19.7123) -> (-14.7321, 21.5167) projected
  arc A48 (-14.7321, 21.5167) -> (-16.0981, 21.8827) centre (-15.5981, 21.0167) ccw projected
  arc A49 (-17.4641, 22.2487) -> (-16.0981, 21.8827) centre (-16.5981, 22.7487) ccw projected
  line L32 (-17.4641, 22.2487) -> (-18.3302, 23.7488) projected
  arc A50 (-11.402, 27.7488) -> (-18.3302, 23.7488) centre (0, 0) ccw projected
  line L33 (-11.402, 27.7488) -> (-10.5359, 26.2487) projected
  arc A51 (-10.9019, 24.8827) -> (-10.5359, 26.2487) centre (-11.4019, 25.7487) ccw projected
  arc A52 (-10.9019, 24.8827) -> (-11.2679, 23.5167) centre (-10.4019, 24.0167) ccw projected
  line L34 (-11.2679, 23.5167) -> (-10.2262, 21.7123) projected
  arc A53 (-2, 23.9165) -> (-10.2262, 21.7123) centre (0, 0) ccw projected
  line L35 (-2, 23.9165) -> (-2, 26) projected
  arc A54 (-2, 26) -> (-3, 27) centre (-3, 26) ccw projected
  arc A55 (-4, 28) -> (-3, 27) centre (-3, 28) ccw projected
  line L36 (-4, 28) -> (-4, 29.7321) projected
  arc A56 (4, 29.7321) -> (-4, 29.7321) centre (0, 0) ccw projected
  line L37 (4, 29.7321) -> (4, 28) projected
  arc A57 (3, 27) -> (4, 28) centre (3, 28) ccw projected
  arc A58 (3, 27) -> (2, 26) centre (3, 26) ccw projected
  line L38 (2, 26) -> (2, 23.9165) projected
  arc A59 (10.2262, 21.7123) -> (2, 23.9165) centre (0, 0) ccw projected
  line L39 (10.2262, 21.7123) -> (11.2679, 23.5167) projected
  arc A60 (11.2679, 23.5167) -> (10.9019, 24.8827) centre (10.4019, 24.0167) ccw projected
  arc A61 (10.5359, 26.2487) -> (10.9019, 24.8827) centre (11.4019, 25.7487) ccw projected
  line L40 (10.5359, 26.2487) -> (11.402, 27.7488) projected
  arc A62 (18.3302, 23.7488) -> (11.402, 27.7488) centre (0, 0) ccw projected
  line L41 (18.3302, 23.7488) -> (17.4641, 22.2487) projected
  arc A63 (16.0981, 21.8827) -> (17.4641, 22.2487) centre (16.5981, 22.7487) ccw projected
  arc A64 (16.0981, 21.8827) -> (14.7321, 21.5167) centre (15.5981, 21.0167) ccw projected
  line L42 (14.7321, 21.5167) -> (13.6903, 19.7123) projected
  arc A65 (19.7123, 13.6903) -> (13.6903, 19.7123) centre (0, 0) ccw projected
  line L43 (19.7123, 13.6903) -> (21.5167, 14.7321) projected
  arc A66 (21.5167, 14.7321) -> (21.8827, 16.0981) centre (21.0167, 15.5981) ccw projected
  arc A67 (22.2487, 17.4641) -> (21.8827, 16.0981) centre (22.7487, 16.5981) ccw projected
  line L44 (22.2487, 17.4641) -> (23.7488, 18.3302) projected
  arc A68 (27.7488, 11.402) -> (23.7488, 18.3302) centre (0, 0) ccw projected
  line L45 (27.7488, 11.402) -> (26.2487, 10.5359) projected
  arc A69 (24.8827, 10.9019) -> (26.2487, 10.5359) centre (25.7487, 11.4019) ccw projected
  arc A70 (24.8827, 10.9019) -> (23.5167, 11.2679) centre (24.0167, 10.4019) ccw projected
  line L46 (23.5167, 11.2679) -> (21.7123, 10.2262) projected
  arc A71 (23.9165, 2) -> (21.7123, 10.2262) centre (0, 0) ccw projected
  line L47 (23.9165, 2) -> (26, 2) projected
  circle A72 centre (0, 0) radius 40 projected
  point P0 (-0.0069, -0.0902)
